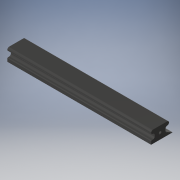
# Autodesk Inventor part: Rail Segment
Saved by Autodesk Inventor 2019 (Build 230136000, 136)
## iProperties
Created: 2020-12-25
Part Number: Rail Segment
Material: Acetal Resin, Black
Document SubType Name: Modeling
Designer: John
Density: 1.425 g/cm^3
Appearance: Smooth - Black
Author: John
Autodesk Inventor part; units mm, degrees
ref_plane "YZ Plane" through (0, 0, 0) normal (1, 0, 0) x (0, 1, 0)
ref_plane "XZ Plane" through (0, 0, 0) normal (0, 1, 0) x (-1, 0, 0)
ref_plane "XY Plane" through (0, 0, 0) normal (0, 0, 1) x (1, 0, 0)
sketch "Sketch1" plane through (0, 0, 0) normal (1, 0, 0) x (0, 1, 0)
  line L0 (-3.175, -15.8752) -> (-3.175, 15.8752)
  line L1 (-3.175, 15.8752) -> (1.9596, -9.7981) construction
  line L2 (3.175, 15.8752) -> (-3.175, -15.8752) construction
  arc A0 (18.3756, 12.7) -> (12.0256, 12.7001) centre (15.2006, 12.7) ccw
  arc A1 (12.0256, -12.7001) -> (18.3756, -12.7) centre (15.2006, -12.7) ccw
  line L3 (8.8506, 9.5252) -> (6.35, 9.5252)
  line L4 (8.8506, -9.5252) -> (5.1346, -9.5252)
  line L5 (15.2006, 12.7) -> (15.2006, -12.7) construction
  line L6 (3.175, 14.6052) -> (3.175, 12.7002)
  arc A2 (8.8506, 9.5252) -> (12.0256, 12.7001) centre (8.8506, 12.7002) ccw
  arc A3 (12.0256, -12.7001) -> (8.8506, -9.5252) centre (8.8506, -12.7002) ccw
  arc A4 (3.175, 12.7002) -> (6.35, 9.5252) centre (6.35, 12.7002) ccw
  arc A5 (5.1346, -9.5252) -> (1.9937, -12.2364) centre (5.1346, -12.7002) ccw
  line L7 (-3.175, -15.8752) -> (-3.175, -22.2252)
  line L8 (1.905, 15.8752) -> (-3.175, 15.8752)
  arc A6 (3.175, 14.6052) -> (1.905, 15.8752) centre (1.905, 14.6052) ccw
  line L9 (18.3756, 12.7) -> (18.3756, -12.7)
  line L10 (1.6475, -13.2791) -> (-3.175, -22.2252)
  arc A7 (1.6475, -13.2791) -> (1.9937, -12.2364) centre (-1.1473, -11.7726) ccw
  line L11 (-3.175, -22.2252) -> (20.4919, -22.2252)
  point P0 (0, 0)
  point P1 (15.2367, 9.5252)
  point P2 (15.2367, -9.5252)
  point P3 (1.9596, -12.7002)
  dimension "d5" = 6.35
  dimension "d8" = 3.175
  dimension "d9" = 6.35
  dimension "d11" = 6.35
  dimension "d12" = 6.35
  dimension "d13" = 1.27
  dimension "d30" = 25.4
  dimension "d31" = 3.175
  constraints: 24 end point, 19 point on circle, 13 tangent, 8 centre point, 6 point on line, 4 equal radius, 2 parallel, 2 perpendicular, 2 vertical, 1 horizontal, 1 midpoint
  measures "d5" diameter of A1
  measures "d8" radius of A2
  measures "d9" distance of L0.start L7.end
  measures "d11" distance between parallel lines of L3 L8
  measures "d12" distance from line of L0.start L4
  measures "d13" radius of A6
  measures "d30" distance of L5.start L5.end
  measures "d31" radius of A7
extrude "Extrusion2" add sketch "Sketch1" along normal mid plane 254
sketch "Sketch5" plane through (127, 0, 0) normal (1, 0, 0) x (0, 0, -1)
  circle A0 centre (0, 7.5946) radius 2.2225
  line L0 (-15.8752, -3.175) -> (22.2252, -3.175) projected
  point P0 (0, 0)
  dimension "d26" = 4.445
  dimension "d27" = 10.7696
  constraints: 1 centre point
  measures "d26" diameter of A0
  measures "d27" distance from line of L0 A0.centre
extrude "Extrusion4" cut sketch "Sketch5" against normal blind 12.7
ref_plane "Work Plane8" through (0, -3.175, 15.8752) normal (0, -1, 0) x (1, 0, 0)
sketch "Sketch7" plane through (0, -3.175, 15.8752) normal (0, -1, 0) x (1, 0, 0)
  line L0 (114.3, -13.6527) -> (114.3, -18.0977) projected
  line L1 (127, -13.6527) -> (127, -18.0977) projected
  line L2 (127, 0) -> (127, -38.1004) projected
  line L3 (127, -15.8752) -> (120.65, -15.8752)
  line L4 (0, -9.5252) -> (120.65, -9.5252)
  line L5 (120.65, -9.5252) -> (120.65, -22.2252)
  line L6 (120.65, -22.2252) -> (0, -22.2252)
  line L7 (0, -22.2252) -> (0, -9.5252)
  line L8 (0, -9.5252) -> (120.65, -22.2252) construction
  line L9 (120.65, -9.5252) -> (0, -22.2252) construction
  point P0 (0, -15.8752)
  point P1 (60.325, -15.8752)
  dimension "d46" = 6.35
  dimension "d47" = 12.7
  dimension "d48" = 120.65
  constraints: 14 end point, 3 midpoint, 2 parallel, 2 perpendicular, 1 horizontal, 1 point on line
  measures "d46" distance of L3.end L3.start
  measures "d47" distance of L4.end L5.end
  measures "d48" distance of L5.end L6.end
extrude "Extrusion7" cut sketch "Sketch7" against normal blind 17.1196
fillet "Fillet2" radius 6.35 2 edges at (60.325, 13.9446, 6.35) (60.325, 13.9446, -6.35)
mirror "Mirror1" about plane through (0, 0, 0) normal (1, 0, 0) of "Extrusion7", "Fillet2", "Extrusion4"
body "Solid2"
